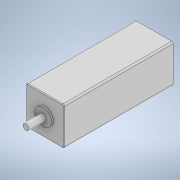
# Autodesk Inventor part: Electric Motor
Saved by Autodesk Inventor 2020 (Build 240168000, 168)
## iProperties
Created: 2020-10-14
Part Number: Electric Motor
Material: Generic
Document SubType Name: Modeling
Designer: jtri402
Density: 1 g/cm^3
Appearance: Default
Author: jtri402
Autodesk Inventor part; units mm, degrees
ref_plane "YZ Plane" through (0, 0, 0) normal (1, 0, 0) x (0, 1, 0)
ref_plane "XZ Plane" through (0, 0, 0) normal (0, 1, 0) x (-1, 0, 0)
ref_plane "XY Plane" through (0, 0, 0) normal (0, 0, 1) x (1, 0, 0)
sketch "Sketch1" plane through (0, 0, 0) normal (0, 0, 1) x (1, 0, 0)
  line L0 (-25, 25) -> (25, 25)
  line L1 (25, 25) -> (25, -25)
  line L2 (25, -25) -> (-25, -25)
  line L3 (-25, -25) -> (-25, 25)
  point P0 (0, 0)
  dimension "d0" = 50
  dimension "d1" = 50
  dimension "d2" = 25
  dimension "d3" = 25
  constraints: 8 end point, 2 parallel, 1 horizontal, 1 perpendicular
  measures "d0" distance of L0.start L0.end
  measures "d1" distance of L0.end L1.end
  measures "d2" distance from line of L3 point (0, 0)
  measures "d3" distance from line of L0 point (0, 0)
extrude "Extrusion1" add sketch "Sketch1" against normal blind 143
sketch "Sketch2" plane through (0, 0, 0) normal (0, 0, 1) x (1, 0, 0)
  circle A0 centre (0, 0) radius 11
  dimension "d7" = 22
  constraints: 1 centre point
  measures "d7" diameter of A0
extrude "Extrusion2" add sketch "Sketch2" along normal blind 2.4
sketch "Sketch3" plane through (0, 0, 2.4) normal (0, 0, 1) x (1, 0, 0)
  circle A0 centre (0, 0) radius 4
  dimension "d10" = 8
  constraints: 1 centre point, 1 coincident
  measures "d10" diameter of A0
extrude "Extrusion3" add sketch "Sketch3" along normal blind 22.5
fillet "Fillet1" radius 2 4 edges at (-25, 25, -71.5) (25, 25, -71.5) (25, -25, -71.5) (-25, -25, -71.5)
fillet "Fillet2" radius 1 8 edges at (-24.4142, 24.4142, 0) (-25, 0, 0) (-24.4142, -24.4142, 0) (0, -25, 0) (24.4142, -24.4142, 0) (25, 0, 0) (24.4142, 24.4142, 0) (0, 25, 0)
body "Solid1"
